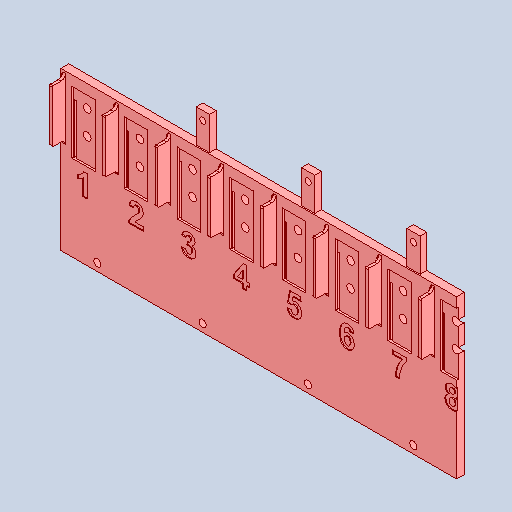
# Autodesk Inventor part: mainPlate
Saved by Autodesk Inventor 2024.3 (Build 283343000, 343)
## iProperties
Created: 2022-10-05
Part Number: mainPlate
Material: Generic
Document SubType Name: Modeling
Designer: Admin
Density: 1 g/cm^3
Appearance: Default(2)
x_d0: 1.000 ul
x_d1: 1.000 ul
x_d2: 1.000 ul
ref:MM:length: 9.750 in
ref:MMC:1: 0.150 in
ref:oring_gap: 0.018 in
ref:fsens:body:4: 0.228 in
ref:fsens:body:6: 0.203 in
ref:fsens:body:2: 0.328 in
ref:fsens:body:5: 1.073 in
ref:fsens:body:1: 1.200 in
ref:fsens:body:3: 0.610 in
ref:fsens:body:7: 0.125 in
ref:fsens:arc_cutout:1: 0.057 in
ref:fsens:arc_cutout:5: 0.550 in
ref:fsens:bottom_grooves:3: 0.940 in
ref:fsens:bottom_grooves:4: 0.058 in
ref:fsens:bottom_grooves:1: 0.155 in
ref:fsens:bottom_grooves:5: 0.500 in
ref:fsens:bottom_grooves:6: 0.040 in
ref:fsens:bottom_grooves:2: 0.473 in
ref:fsens:headerpins:2: 0.025 in
ref:fsens:headerpins:3: 0.100 in
ref:fsens:headerpins:4: 0.100 in
ref:fsens:headerpins:1: 0.025 in
ref:fsens:headerpins:5: 0.001 in
ref:fsens:arc_cutout:3: 0.325 in
ref:fsens:arc_cutout:4: 0.207 in
headerpins:extra_top_space: 0.125 in
headerpins:distance_to_clear_MM_and_MMC: 0.293 in
a_MP_thickness: 0.180 in
x_e0: 0.00 deg
x_e2: 0.00 deg
headerpins:wiggleroom:vertical: 0.491 in
bottom_groove:extra_top_space: 0.025 in
bottom_groove:distance_to_clear_MM_and_MMC: 0.293 in
bottom_groove:wiggleroom:vertical: 0.100 in
bottom_groove:extra_side_space_back: 0.010 in
fsens:bottom_groove:depth: 0.045 in
fsens:hole_diameter: 0.175 in
headerpins:extra_side_space: 0.005 in
p_num_patterns: 8.000 ul
p_pattern_spacing: 1.200 in
ref:fsens:arc_cutout:2: 0.110 in
ref:fsens:body:6:2: 0.203 in
ref:fsens:body:5:2: 1.073 in
ref:fsens:body:3:2: 0.610 in
ref:fsens:bottom_grooves:3:2: 0.940 in
ref:fsens:bottom_grooves:1:2: 0.155 in
ref:fsens:bottom_grooves:6:2: 0.040 in
ref:fsens:bottom_grooves:2:2: 0.473 in
bottom_groove:to_side: 0.250 in
ref:fsens_btm_groove_8th_one: 8.400 in
bottom_groove:to_side:2: 0.010 in
ref_440_throughhole: 0.165 in
MMscrews:to_top: 0.200 in
d133: 0.180 in
x_e3: 0.00 deg
MMscrews:through_hole:diameter: 0.140 in
MMscrews_popup_width: 0.300 in
ref:MMC:height: 0.150 in
ref:MM:width: 1.100 in
ref:MM:height: 0.800 in
d148: 0.018 in
MMC_to_top_of_MP: 0.030 in
d168: 0.029 in
d171: 0.029 in
x_e4: 0.00 deg
headerpins_space_for_PCB_female_headers: 0.150 in
headerpins:cutout_depth: 0.100 in
bottom_groove:extra_side_space_front: 0.020 in
fsens:front_wall:width: 0.085 in
fsens:front_wall:height: 0.300 in
x_e: 0.00 deg
d219: 0.025 in
d220: 0.025 in
d222: 0.100 in
d223: 0.025 in
numbers_width: 0.300 in
numbers_height: 0.500 in
numbers_space_between: 1.200 in
numbers_: 0.100 in
d244: 0.020 in
d245: 0.00 deg
d246: 0.300 in
d247: 0.500 in
d248: 0.100 in
d281: 0.020 in
d285: 0.165 in
d292: 2.400 in
d293: 2.400 in
d294: 2.400 in
d295: 3.975 in
d296: 0.025 in
d297: 0.175 in
d300: 9.016 in
d302: 0.00 deg
d303: 0.165 in
distance_to_clear_MM_and_MMC: 0.293 in
threadInsert_440:diameter: 0.175 in
bottom_groove:to_top: 0.230 in
d170: 0.035 in
a_mainManifold:x:length: 9.750 in
flowSensor:hole_insert:depth: 0.125 in
a_mainManifoldCover:y:height: 0.150 in
dsheet:side:z:1: 0.610 in
dsheet:front:x:1: 1.200 in
dsheet:front:x:4: 0.025 in
dsheet:front:x:2: 0.940 in
dsheet:front:x:3:1: 0.100 in
dsheet:top:x:3: 0.250 in
dsheet:top:x:4: 0.300 in
dsheet:top:x:2: 0.110 in
z_width: 0.328 in
headerpins_depth: 0.025 in
x_d47: 0.058 in
x_d51: 0.155 in
dsheet:front:x:3:2: 0.100 in
x_d53: 0.473 in
d55: 0.500 in
dsheet:top:x:1: 2.145 in
d64: 0.228 in
dsheet:side:z:4: 0.325 in
d65: 0.203 in
distance_between_MFCs: 1.200 in
a_mainManifold:y:height: 0.800 in
a_mainManifold:z:width: 1.100 in
Author: Admin
Autodesk Inventor part; units mm, degrees
ref_plane "YZ Plane" through (0, 0, 0) normal (1, 0, 0) x (0, 1, 0)
ref_plane "XZ Plane" through (0, 0, 0) normal (0, 1, 0) x (-1, 0, 0)
derived "main_manifold_8v_v02.ipt"
sketch "Sketch:MM: main inlet" plane through (0, 0, 0) normal (1, 0, 0) x (0, 1, 0)
  line L0 (20.32, 0) -> (0, 0)
  line L1 (0, 0) -> (0, -27.94)
  line L2 (0, -27.94) -> (20.32, -27.94)
  line L3 (20.32, -27.94) -> (20.32, 0)
  point P0 (13.97, -15.24)
sketch "Sketch:MM: prop valves" plane through (0, 0, -27.94) normal (0, 0, -1) x (-1, 0, 0)
  line L0 (-16.9926, 9.0678) -> (-24.9174, 9.0678) construction
  line L1 (-47.4726, 9.0678) -> (-55.3974, 9.0678) construction
  line L2 (-77.9526, 9.0678) -> (-85.8774, 9.0678) construction
  line L3 (-108.4326, 9.0678) -> (-116.3574, 9.0678) construction
  line L4 (-138.9126, 9.0678) -> (-146.8374, 9.0678) construction
  line L5 (-169.3926, 9.0678) -> (-177.3174, 9.0678) construction
  line L6 (-199.8726, 9.0678) -> (-207.7974, 9.0678) construction
  line L7 (-230.3526, 9.0678) -> (-238.2774, 9.0678) construction
  line L8 (-47.4726, 9.0678) -> (-51.435, 5.3848) construction
  line L9 (-16.9926, 9.0678) -> (-20.955, 5.3848) construction
  line L10 (-77.9526, 9.0678) -> (-81.915, 5.3848) construction
  line L11 (-169.3926, 9.0678) -> (-173.355, 5.3848) construction
  line L12 (-199.8726, 9.0678) -> (-203.835, 5.3848) construction
  line L13 (-230.3526, 9.0678) -> (-234.315, 5.3848) construction
  line L14 (-138.9126, 9.0678) -> (-142.875, 5.3848) construction
  line L15 (-108.4326, 9.0678) -> (-112.395, 5.3848) construction
  line L16 (-20.955, 12.5222) -> (-51.435, 12.5222) construction
  line L17 (-51.435, 12.5222) -> (-81.915, 12.5222) construction
  line L18 (-81.915, 12.5222) -> (-112.395, 12.5222) construction
  line L19 (-112.395, 12.5222) -> (-142.875, 12.5222) construction
  line L20 (-142.875, 12.5222) -> (-173.355, 12.5222) construction
  line L21 (-173.355, 12.5222) -> (-203.835, 12.5222) construction
  line L22 (-203.835, 12.5222) -> (-234.315, 12.5222) construction
  point P0 (0, 0)
  point P1 (0, 13.97)
sketch "Sketch:MM: prop valve cutout" plane through (0, 0, 0) normal (1, 0, 0) x (0, 1, 0)
  line L0 (20.32, -27.94) -> (20.32, 0)
  line L1 (0, -27.94) -> (20.32, -27.94)
  line L2 (20.32, -25.781) -> (16.256, -25.781)
  line L3 (16.256, -25.781) -> (16.256, -27.94)
  point P0 (0, 0)
  point P1 (12.5222, -27.94)
sketch "Sketch:MM: flow sensor" plane through (0, 0, -27.94) normal (0, -1, 0) x (1, 0, 0)
  line L0 (19.2278, 23.241) -> (22.6822, 23.241)
  line L1 (49.7078, 23.241) -> (53.1622, 23.241)
  line L2 (110.6678, 23.241) -> (114.1222, 23.241)
  line L3 (80.1878, 23.241) -> (83.6422, 23.241)
  line L4 (141.1478, 23.241) -> (144.6022, 23.241)
  line L5 (171.6278, 23.241) -> (175.0822, 23.241)
  line L6 (202.1078, 23.241) -> (205.5622, 23.241)
  line L7 (232.5878, 23.241) -> (236.0422, 23.241)
  line L8 (0, 27.94) -> (247.65, 27.94)
  point P0 (20.955, 23.241)
  point P1 (51.435, 23.241)
  point P2 (51.435, 23.241)
  point P3 (20.955, 23.241)
  point P4 (81.915, 23.241)
  point P5 (112.395, 23.241)
  point P6 (81.915, 23.241)
  point P7 (112.395, 23.241)
  point P8 (142.875, 23.241)
  point P9 (173.355, 23.241)
  point P10 (203.835, 23.241)
  point P11 (234.315, 23.241)
  point P12 (142.875, 23.241)
  point P13 (173.355, 23.241)
  point P14 (203.835, 23.241)
  point P15 (234.315, 23.241)
sketch "Sketch:MM: MMC screws" plane through (0, 20.32, 0) normal (0, 1, 0) x (1, 0, 0)
  line L0 (0, 0) -> (0, 27.94)
  line L1 (43.815, 4.699) -> (59.055, 4.699) construction
  line L2 (0, 0) -> (247.65, 0)
  line L3 (13.335, 4.699) -> (28.575, 4.699) construction
  line L4 (74.295, 4.699) -> (89.535, 4.699) construction
  line L5 (104.775, 4.699) -> (120.015, 4.699) construction
  line L6 (135.255, 4.699) -> (150.495, 4.699) construction
  line L7 (165.735, 4.699) -> (180.975, 4.699) construction
  line L8 (196.215, 4.699) -> (211.455, 4.699) construction
  line L9 (226.695, 4.699) -> (241.935, 4.699) construction
  point P0 (20.955, 4.699)
  point P1 (112.395, 4.699)
  point P2 (51.435, 4.699)
  point P3 (81.915, 4.699)
  point P4 (0, 25.781)
  point P5 (0, 25.781)
  point P6 (0, 25.781)
  point P7 (142.875, 4.699)
  point P8 (173.355, 4.699)
  point P9 (203.835, 4.699)
  point P10 (234.315, 4.699)
  point P11 (20.955, 4.699)
  point P12 (51.435, 4.699)
  point P13 (81.915, 4.699)
  point P14 (112.395, 4.699)
  point P15 (142.875, 4.699)
  point P16 (173.355, 4.699)
  point P17 (203.835, 4.699)
  point P18 (234.315, 4.699)
sketch "Sketch:MM: MP screws" plane through (0, 0, 0) normal (0, 0, 1) x (1, 0, 0)
  point P0 (0, 0)
  point P1 (5.08, 9.0678)
  point P2 (218.44, 9.0678)
  point P3 (96.52, 9.0678)
  point P4 (157.48, 9.0678)
sketch "Sketch:MM: mounting screws:1" plane through (0, 0, 0) normal (-1, 0, 0) x (0, 0, 1)
  line L0 (-27.94, 0) -> (-27.94, 16.256)
  line L1 (-21.59, 5.08) -> (-8.89, 5.08) construction
  point P0 (0, 0)
  point P1 (-15.24, 13.97)
  point P2 (-15.24, 5.08)
sketch "Sketch:MM: mounting screws:2" plane through (247.65, 0, 0) normal (1, 0, 0) x (0, 0, -1)
  point P0 (0, 0)
  point P1 (21.59, 5.08)
  point P2 (8.89, 5.08)
ref_plane "MM front face" through (0, 0, 0) normal (0, 0, 1) x (1, 0, 0)
derived "main_manifold_cover_1v_v02.ipt"
sketch "Sketch:MMC: base" plane through (0, 0, 0) normal (0, 1, 0) x (-1, 0, 0)
  line L0 (-9.779, -9.398) -> (-32.131, -9.398)
  line L1 (-32.131, -9.398) -> (-32.131, 0)
  line L2 (-32.131, 0) -> (-9.779, 0)
  line L3 (-9.779, 0) -> (-9.779, -9.398)
  point P0 (0, 0)
  point P1 (-43.815, -4.699)
  point P2 (-9.779, -4.699)
  point P3 (-13.335, -4.699)
  point P4 (-28.575, -4.699)
derived "Honeywell3000.ipt"
sketch "Sketch:ref: assembly:XY" plane through (0, 0, 0) normal (0, 0, 1) x (1, 0, 0)
  line L0 (0, 20.32) -> (0, 0) projected
  line L1 (0, 20.32) -> (247.65, 20.32)
  line L2 (247.65, 20.32) -> (247.65, 0)
  line L3 (247.65, 0) -> (0, 0)
  line L4 (9.779, 0) -> (32.131, 0) projected
  line L5 (9.779, -0.4572) -> (32.131, -0.4572)
  line L6 (32.131, -0.4572) -> (32.131, -4.2672)
  line L7 (32.131, -4.2672) -> (9.779, -4.2672)
  line L8 (9.779, -4.2672) -> (9.779, -0.4572)
  line L9 (18.0536, 3.175) -> (23.8564, 3.175)
  line L10 (23.8564, 3.175) -> (23.8564, -8.8265)
  line L11 (23.8564, -8.8265) -> (18.0536, -8.8265)
  line L12 (18.0536, -8.8265) -> (18.0536, 3.175)
  line L13 (17.7869, -8.8265) -> (26.1181, -8.8265)
  line L14 (26.1181, -8.8265) -> (26.1181, -39.3065)
  line L15 (26.1181, -39.3065) -> (17.7869, -39.3065)
  line L16 (17.7869, -39.3065) -> (17.7869, -8.8265)
  line L17 (26.1181, -8.8265) -> (33.2809, -8.8265)
  line L18 (33.2809, -8.8265) -> (33.2809, -39.3065)
  line L19 (33.2809, -39.3065) -> (26.1181, -39.3065)
  arc A0 (30.6647, -17.2745) -> (27.7691, -17.2745) centre (29.2169, -17.2745) ccw
  arc A1 (27.7691, -20.0685) -> (30.6647, -20.0685) centre (29.2169, -20.0685) ccw
  line L20 (27.7691, -20.0685) -> (27.7691, -17.2745)
  line L21 (30.6647, -20.0685) -> (30.6647, -17.2745)
  arc A2 (30.6647, -31.2445) -> (27.7691, -31.2445) centre (29.2169, -31.2445) ccw
  arc A3 (27.7691, -34.0385) -> (30.6647, -34.0385) centre (29.2169, -34.0385) ccw
  line L22 (27.7691, -34.0385) -> (27.7691, -31.2445)
  line L23 (30.6647, -34.0385) -> (30.6647, -31.2445)
  line L24 (29.2169, -17.2745) -> (29.2169, -20.0685) construction
  line L25 (29.2169, -31.2445) -> (29.2169, -34.0385) construction
  line L26 (21.971, -11.4935) -> (34.671, -11.4935)
  line L27 (34.671, -11.4935) -> (34.671, -12.9667)
  line L28 (34.671, -12.9667) -> (21.971, -12.9667)
  line L29 (21.971, -12.9667) -> (21.971, -11.4935)
  line L30 (21.971, -24.8412) -> (34.671, -24.8412)
  line L31 (34.671, -24.8412) -> (34.671, -26.3144)
  line L32 (34.671, -26.3144) -> (21.971, -26.3144)
  line L33 (21.971, -26.3144) -> (21.971, -24.8412)
  line L34 (21.971, -36.8427) -> (34.671, -36.8427)
  line L35 (34.671, -36.8427) -> (34.671, -35.3695)
  line L36 (34.671, -35.3695) -> (21.971, -35.3695)
  line L37 (21.971, -35.3695) -> (21.971, -36.8427)
  line L38 (21.971, -21.209) -> (22.606, -21.209)
  line L39 (22.606, -21.209) -> (22.606, -21.844)
  line L40 (22.606, -21.844) -> (21.971, -21.844)
  line L41 (21.971, -21.844) -> (21.971, -21.209)
  line L42 (21.971, -23.749) -> (22.606, -23.749)
  line L43 (22.606, -23.749) -> (22.606, -24.384)
  line L44 (22.606, -24.384) -> (21.971, -24.384)
  line L45 (21.971, -24.384) -> (21.971, -23.749)
  line L46 (21.971, -26.289) -> (22.606, -26.289)
  line L47 (22.606, -26.289) -> (22.606, -26.924)
  line L48 (22.606, -26.924) -> (21.971, -26.924)
  line L49 (21.971, -26.924) -> (21.971, -26.289)
  line L50 (231.4136, 3.175) -> (237.2164, 3.175)
  line L51 (237.2164, 3.175) -> (237.2164, -8.8265)
  line L52 (237.2164, -8.8265) -> (231.4136, -8.8265)
  line L53 (231.4136, -8.8265) -> (231.4136, 3.175)
  line L54 (231.1469, -8.8265) -> (239.4781, -8.8265)
  line L55 (239.4781, -8.8265) -> (239.4781, -39.3065)
  line L56 (239.4781, -39.3065) -> (231.1469, -39.3065)
  line L57 (231.1469, -39.3065) -> (231.1469, -8.8265)
  line L58 (239.4781, -8.8265) -> (246.6409, -8.8265)
  line L59 (246.6409, -8.8265) -> (246.6409, -39.3065)
  line L60 (246.6409, -39.3065) -> (239.4781, -39.3065)
  line L61 (235.331, -11.4935) -> (248.031, -11.4935)
  line L62 (248.031, -11.4935) -> (248.031, -12.9667)
  line L63 (248.031, -12.9667) -> (235.331, -12.9667)
  line L64 (235.331, -12.9667) -> (235.331, -11.4935)
  line L65 (235.331, -24.8412) -> (248.031, -24.8412)
  line L66 (248.031, -24.8412) -> (248.031, -26.3144)
  line L67 (248.031, -26.3144) -> (235.331, -26.3144)
  line L68 (235.331, -26.3144) -> (235.331, -24.8412)
  line L69 (235.331, -36.8427) -> (248.031, -36.8427)
  line L70 (248.031, -36.8427) -> (248.031, -35.3695)
  line L71 (248.031, -35.3695) -> (235.331, -35.3695)
  line L72 (235.331, -35.3695) -> (235.331, -36.8427)
  point P0 (20.955, 3.175)
  point P1 (20.955, 3.175)
  point P2 (17.7869, -24.0665)
  point P3 (17.7869, -24.0665)
  point P4 (20.955, 0)
  point P5 (29.2169, -32.6415)
  point P6 (29.2169, -18.6715)
  point P7 (29.2169, -18.6715)
  point P8 (34.671, -36.1061)
  point P9 (34.671, -36.1061)
  point P10 (34.671, -12.2301)
  point P11 (34.671, -12.2301)
  point P12 (22.606, -21.5265)
  point P13 (22.606, -24.0665)
  point P14 (22.606, -21.5265)
  point P15 (22.606, -24.0665)
  point P16 (22.606, -26.6065)
  point P17 (22.606, -26.6065)
  point P18 (234.315, 3.175)
  point P19 (234.315, 3.175)
  point P20 (231.1469, -24.0665)
  point P21 (231.1469, -24.0665)
  point P22 (248.031, -36.1061)
  point P23 (248.031, -36.1061)
  point P24 (248.031, -12.2301)
  point P25 (248.031, -12.2301)
  point P26 (234.315, 0)
  constraints: 142 end point, 44 perpendicular, 21 equal length, 16 coincident, 15 collinear, 14 vertical alignment, 13 midpoint, 8 parallel, 8 point on circle, 8 tangent, 6 horizontal, 5 horizontal alignment, 4 centre point, 4 point on line, 3 equal radius, 2 vertical, 10 other
sketch "x_Sketch:ref: assembly:YZ" plane through (0, 0, 0) normal (1, 0, 0) x (0, 1, 0)
  line L0 (-0.4572, 27.2034) -> (-4.2672, 27.2034)
  line L1 (-4.2672, 27.2034) -> (-4.2672, 17.8054)
  line L2 (-4.2672, 17.8054) -> (-0.4572, 17.8054)
  line L3 (-0.4572, 17.8054) -> (-0.4572, 27.2034)
  line L4 (0, -9.398) -> (0, 0) construction
  line L5 (20.32, 27.2034) -> (0, 27.2034)
  line L6 (0, 27.2034) -> (0, -0.7366)
  line L7 (0, -0.7366) -> (20.32, -0.7366)
  line L8 (20.32, -0.7366) -> (20.32, 27.2034)
  point P0 (0, 0)
  dimension "d148" = 0.4572
  dimension "d168" = 0.7366
  constraints: 16 end point, 6 perpendicular, 2 horizontal, 2 horizontal alignment, 1 collinear, 1 parallel, 1 point on line, 1 vertical alignment
  measures "d148" distance between parallel lines of L3 L6
  measures "d168" distance from line of point (0, 0) L7
sketch "Sketch:MP:fSens header pins" plane through (0, 0, 0) normal (0, 0, 1) x (1, 0, 0)
  line L0 (17.7869, -39.3065) -> (17.7869, -8.8265) construction
  line L1 (33.2809, -8.8265) -> (33.2809, -39.3065) construction
  line L2 (26.1181, -39.3065) -> (17.7869, -39.3065) construction
  line L3 (33.2809, -39.3065) -> (26.1181, -39.3065) construction
  line L4 (26.1181, -8.8265) -> (33.2809, -8.8265) construction
  line L5 (17.7869, -8.8265) -> (26.1181, -8.8265) construction
  line L6 (30.6647, -20.0685) -> (30.6647, -17.2745) construction
  arc A0 (30.6647, -17.2745) -> (27.7691, -17.2745) centre (29.2169, -17.2745) ccw construction
  line L7 (27.7691, -20.0685) -> (27.7691, -17.2745) construction
  arc A1 (27.7691, -20.0685) -> (30.6647, -20.0685) centre (29.2169, -20.0685) ccw construction
  arc A2 (30.6647, -31.2445) -> (27.7691, -31.2445) centre (29.2169, -31.2445) ccw construction
  line L8 (30.6647, -34.0385) -> (30.6647, -31.2445) construction
  arc A3 (27.7691, -34.0385) -> (30.6647, -34.0385) centre (29.2169, -34.0385) ccw construction
  line L9 (27.7691, -34.0385) -> (27.7691, -31.2445) construction
  line L10 (22.606, -26.924) -> (21.971, -26.924) construction
  line L11 (21.971, -26.924) -> (21.971, -26.289) construction
  line L12 (22.606, -26.289) -> (22.606, -26.924) construction
  line L13 (21.971, -26.289) -> (22.606, -26.289) construction
  line L14 (22.606, -24.384) -> (21.971, -24.384) construction
  line L15 (22.606, -23.749) -> (22.606, -24.384) construction
  line L16 (21.971, -24.384) -> (21.971, -23.749) construction
  line L17 (21.971, -23.749) -> (22.606, -23.749) construction
  line L18 (22.606, -21.844) -> (21.971, -21.844) construction
  line L19 (22.606, -21.209) -> (22.606, -21.844) construction
  line L20 (21.971, -21.844) -> (21.971, -21.209) construction
  line L21 (21.971, -21.209) -> (22.606, -21.209) construction
  line L22 (21.971, -11.4935) -> (34.671, -11.4935) construction
  line L23 (21.971, -12.9667) -> (21.971, -11.4935) construction
  line L24 (34.671, -12.9667) -> (21.971, -12.9667) construction
  line L25 (34.671, -11.4935) -> (34.671, -12.9667) construction
  line L26 (34.671, -26.3144) -> (21.971, -26.3144) construction
  line L27 (21.971, -24.8412) -> (34.671, -24.8412) construction
  line L28 (34.671, -24.8412) -> (34.671, -26.3144) construction
  line L29 (21.971, -26.3144) -> (21.971, -24.8412) construction
  line L30 (34.671, -35.3695) -> (21.971, -35.3695) construction
  line L31 (21.971, -35.3695) -> (21.971, -36.8427) construction
  line L32 (21.971, -36.8427) -> (34.671, -36.8427) construction
  line L33 (34.671, -36.8427) -> (34.671, -35.3695) construction
  line L34 (21.844, -18.034) -> (22.733, -18.034)
  line L35 (22.733, -18.034) -> (22.733, -46.8249)
  line L36 (22.733, -46.8249) -> (21.844, -46.8249)
  line L37 (21.844, -46.8249) -> (21.844, -18.034)
  line L38 (22.733, -34.3662) -> (21.844, -34.3662) construction
  line L39 (20.3835, -18.034) -> (24.1935, -18.034)
  line L40 (24.1935, -18.034) -> (24.1935, -46.8249)
  line L41 (24.1935, -46.8249) -> (20.3835, -46.8249)
  line L42 (20.3835, -46.8249) -> (20.3835, -18.034)
  point P0 (0, 0)
  point P1 (22.2885, -18.034)
  point P2 (22.2885, -21.209)
  point P3 (22.2885, -18.034)
  dimension "headerpins_space_for_PCB_female_headers" = 3.81
  constraints: 18 end point, 7 perpendicular, 4 parallel, 3 midpoint, 2 collinear, 2 point on line, 1 coincident, 1 horizontal, 1 vertical alignment
  measures "headerpins_space_for_PCB_female_headers" distance of L39.start L39.end
sketch "Sketch:MP:fSens bottom groove" plane through (0, 0, 0) normal (0, 0, 1) x (1, 0, 0)
  line L0 (21.971, -11.4935) -> (34.671, -11.4935) construction
  line L1 (21.971, -12.9667) -> (21.971, -11.4935) construction
  line L2 (34.671, -12.9667) -> (21.971, -12.9667) construction
  line L3 (34.671, -11.4935) -> (34.671, -12.9667) construction
  line L4 (34.671, -24.8412) -> (34.671, -26.3144) construction
  line L5 (21.971, -24.8412) -> (34.671, -24.8412) construction
  line L6 (34.671, -26.3144) -> (21.971, -26.3144) construction
  line L7 (21.971, -26.3144) -> (21.971, -24.8412) construction
  line L8 (34.671, -35.3695) -> (21.971, -35.3695) construction
  line L9 (34.671, -36.8427) -> (34.671, -35.3695) construction
  line L10 (21.971, -36.8427) -> (34.671, -36.8427) construction
  line L11 (21.971, -35.3695) -> (21.971, -36.8427) construction
  line L12 (21.463, -10.8585) -> (34.925, -10.8585)
  line L13 (34.925, -10.8585) -> (34.925, -46.8249)
  line L14 (34.925, -46.8249) -> (21.463, -46.8249)
  line L15 (21.463, -46.8249) -> (21.463, -10.8585)
  line L16 (34.925, -44.2849) -> (21.463, -44.2849) construction
  line L17 (22.733, -18.034) -> (22.733, -46.8249) construction
  line L18 (21.844, -18.034) -> (22.733, -18.034) construction
  line L19 (21.844, -46.8249) -> (21.844, -18.034) construction
  line L20 (22.733, -46.8249) -> (21.844, -46.8249) construction
  point P0 (0, 0)
  point P1 (28.321, -11.4935)
  point P2 (28.194, -10.8585)
  constraints: 8 end point, 4 parallel, 3 horizontal, 2 midpoint, 2 perpendicular, 1 point on line, 1 vertical, 4 other
sketch "Sketch:MP:fSens front wall" plane through (0, 0, 0) normal (0, 0, 1) x (1, 0, 0)
  line L0 (15.6279, -8.8265) -> (17.7869, -8.8265)
  line L1 (17.7869, -8.8265) -> (17.7869, -39.3065)
  line L2 (17.7869, -39.3065) -> (15.6279, -39.3065)
  line L3 (15.6279, -39.3065) -> (15.6279, -8.8265)
  line L4 (17.7869, -39.3065) -> (17.7869, -8.8265) construction
  line L5 (17.7869, -8.8265) -> (26.1181, -8.8265) construction
  line L6 (26.1181, -39.3065) -> (17.7869, -39.3065) construction
  point P0 (0, 0)
  constraints: 8 end point, 3 collinear, 2 parallel, 1 horizontal, 1 horizontal alignment, 1 perpendicular
sketch "Sketch:MP: VH holes" plane through (0, 0, 0) normal (0, 0, 1) x (1, 0, 0)
  line L0 (36.195, -91.8972) -> (97.155, -91.8972)
  line L1 (97.155, -91.8972) -> (158.115, -91.8972)
  line L2 (158.115, -91.8972) -> (219.075, -91.8972)
  point P0 (0, 0)
  point P1 (5.08, 9.0678)
  point P2 (96.52, 9.0678)
  point P3 (157.48, 9.0678)
  point P4 (218.44, 9.0678)
  dimension "d292" = 60.96
  dimension "d293" = 60.96
  dimension "d294" = 60.96
  dimension "d295" = 100.965
  dimension "d296" = 0.635
  constraints: 6 end point, 4 coincident, 3 horizontal alignment
  measures "d292" distance of L0.start L0.end
  measures "d293" distance of L0.end L1.end
  measures "d294" distance of L1.end L2.end
  measures "d295" vertical distance of point (219.075, -91.897) point (218.44, 9.068)
  measures "d296" horizontal distance of point (219.075, -91.897) point (218.44, 9.068)
sketch "Sketch:MP:base" plane through (0, 0, 0) normal (0, 0, 1) x (1, 0, 0)
  line L0 (15.113, -5.0292) -> (248.539, -5.0292)
  line L1 (248.539, -5.0292) -> (248.539, -96.3422)
  line L2 (248.539, -96.3422) -> (15.113, -96.3422)
  line L3 (15.113, -96.3422) -> (15.113, -5.0292)
  line L4 (21.463, -10.8585) -> (34.925, -10.8585) construction
  line L5 (21.463, -46.8249) -> (21.463, -10.8585) construction
  line L6 (34.925, -10.8585) -> (34.925, -46.8249) construction
  line L7 (34.925, -46.8249) -> (21.463, -46.8249) construction
  line L8 (234.823, -10.8585) -> (248.285, -10.8585) construction
  line L9 (248.285, -10.8585) -> (248.285, -46.8249) construction
  line L10 (248.285, -46.8249) -> (234.823, -46.8249) construction
  line L11 (234.823, -46.8249) -> (234.823, -10.8585) construction
  line L12 (247.65, 0) -> (0, 0) construction
  line L13 (32.131, -4.2672) -> (9.779, -4.2672) construction
  line L14 (9.779, -4.2672) -> (9.779, -0.4572) construction
  line L15 (9.779, -0.4572) -> (32.131, -0.4572) construction
  line L16 (32.131, -0.4572) -> (32.131, -4.2672) construction
  point P0 (36.195, -91.8972)
  point P1 (97.155, -91.8972)
  point P2 (158.115, -91.8972)
  point P3 (219.075, -91.8972)
  dimension "MMC_to_top_of_MP" = 0.762
  dimension "d170" = 0.889
  dimension "d297" = 4.445
  constraints: 16 end point, 4 equal length, 4 parallel, 2 perpendicular, 1 collinear
  measures "MMC_to_top_of_MP" distance between parallel lines of L0 L13
  measures "d170" distance from line of L1 L12.start
  measures "d297" distance from line of L2 point (36.195, -91.897)
sketch "Sketch:MP: MM screws" plane through (0, 0, 0) normal (0, 0, 1) x (1, 0, 0)
  line L0 (0, 20.32) -> (247.65, 20.32) construction
  line L1 (247.65, 20.32) -> (247.65, 0) construction
  line L2 (0, 20.32) -> (0, 0) construction
  line L3 (247.65, 0) -> (0, 0) construction
  line L4 (15.113, -96.3422) -> (15.113, -5.0292) projected
  line L5 (15.113, -5.0292) -> (248.539, -5.0292) projected
  line L6 (248.539, -5.0292) -> (248.539, -96.3422) projected
  line L7 (92.71, -5.0292) -> (92.71, 14.1478)
  line L8 (92.71, 14.1478) -> (100.33, 14.1478)
  line L9 (100.33, 14.1478) -> (100.33, -5.0292)
  line L10 (153.67, -5.0292) -> (153.67, 14.1478)
  line L11 (153.67, 14.1478) -> (161.29, 14.1478)
  line L12 (161.29, 14.1478) -> (161.29, -5.0292)
  line L13 (214.63, -5.0292) -> (214.63, 14.1478)
  line L14 (214.63, 14.1478) -> (222.25, 14.1478)
  line L15 (222.25, 14.1478) -> (222.25, -5.0292)
  circle A0 centre (96.52, 9.0678) radius 2.0955 construction
  point P0 (5.08, 9.0678)
  point P1 (157.48, 9.0678)
  point P2 (218.44, 9.0678)
  point P3 (96.52, 14.1478)
  point P4 (157.48, 14.1478)
  point P5 (218.44, 14.1478)
  dimension "ref_440_throughhole" = 4.191
  dimension "MMscrews_popup_width" = 7.62
  constraints: 18 end point, 9 perpendicular, 6 point on line, 4 collinear, 3 midpoint, 3 vertical alignment, 1 centre point, 1 coincident, 1 other
  measures "ref_440_throughhole" diameter of A0
  measures "MMscrews_popup_width" distance of L7.end L8.end
sketch "Sketch:MP:numbers_front" plane through (0, 0, 0) normal (0, 0, 1) x (1, 0, 0)
  line L0 (24.384, -50.1583) -> (32.004, -50.1583) construction
  line L1 (32.004, -50.1583) -> (32.004, -62.8583) construction
  line L2 (32.004, -62.8583) -> (24.384, -62.8583) construction
  line L3 (24.384, -62.8583) -> (24.384, -50.1583) construction
  line L4 (54.864, -50.1583) -> (62.484, -50.1583) construction
  line L5 (62.484, -50.1583) -> (62.484, -62.8583) construction
  line L6 (62.484, -62.8583) -> (54.864, -62.8583) construction
  line L7 (54.864, -62.8583) -> (54.864, -50.1583) construction
  line L8 (85.344, -50.1583) -> (92.964, -50.1583) construction
  line L9 (92.964, -50.1583) -> (92.964, -62.8583) construction
  line L10 (92.964, -62.8583) -> (85.344, -62.8583) construction
  line L11 (85.344, -62.8583) -> (85.344, -50.1583) construction
  line L12 (115.824, -50.1583) -> (123.444, -50.1583) construction
  line L13 (123.444, -50.1583) -> (123.444, -62.8583) construction
  line L14 (123.444, -62.8583) -> (115.824, -62.8583) construction
  line L15 (115.824, -62.8583) -> (115.824, -50.1583) construction
  line L16 (146.304, -50.1583) -> (153.924, -50.1583) construction
  line L17 (153.924, -50.1583) -> (153.924, -62.8583) construction
  line L18 (153.924, -62.8583) -> (146.304, -62.8583) construction
  line L19 (146.304, -62.8583) -> (146.304, -50.1583) construction
  line L20 (176.784, -50.1583) -> (184.404, -50.1583) construction
  line L21 (184.404, -50.1583) -> (184.404, -62.8583) construction
  line L22 (184.404, -62.8583) -> (176.784, -62.8583) construction
  line L23 (176.784, -62.8583) -> (176.784, -50.1583) construction
  line L24 (207.264, -50.1583) -> (214.884, -50.1583) construction
  line L25 (214.884, -50.1583) -> (214.884, -62.8583) construction
  line L26 (214.884, -62.8583) -> (207.264, -62.8583) construction
  line L27 (207.264, -62.8583) -> (207.264, -50.1583) construction
  line L28 (237.744, -50.1583) -> (245.364, -50.1583) construction
  line L29 (245.364, -50.1583) -> (245.364, -62.8583) construction
  line L30 (245.364, -62.8583) -> (237.744, -62.8583) construction
  line L31 (237.744, -62.8583) -> (237.744, -50.1583) construction
  line L32 (28.194, -65.3983) -> (58.674, -65.3983) construction
  line L33 (58.674, -65.3983) -> (89.154, -65.3983) construction
  line L34 (89.154, -65.3983) -> (119.634, -65.3983) construction
  line L35 (119.634, -65.3983) -> (150.114, -65.3983) construction
  line L36 (150.114, -65.3983) -> (180.594, -65.3983) construction
  line L37 (180.594, -65.3983) -> (211.074, -65.3983) construction
  line L38 (211.074, -65.3983) -> (241.554, -65.3983) construction
  line L39 (21.463, -10.8585) -> (34.925, -10.8585) construction
  line L40 (34.925, -10.8585) -> (34.925, -46.8249) construction
  line L41 (21.463, -46.8249) -> (21.463, -10.8585) construction
  line L42 (34.925, -46.8249) -> (21.463, -46.8249) construction
  line L43 (30.251, -62.9067) -> (27.8116, -62.9067)
  line L44 (27.8116, -62.9067) -> (27.8116, -53.7398)
  spline S0 degree 2 poles (27.8116, -53.7398) (26.4758, -54.9789) (24.6657, -55.579) knots 0 0 0 1 1 1
  line L45 (24.6657, -55.579) -> (24.6657, -53.372)
  spline S1 degree 2 poles (24.6657, -53.372) (25.624, -53.0622) (27.86, -51.3199) (28.2763, -50.1583) knots 0 0 0 1 2 2 2
  line L46 (28.2763, -50.1583) -> (30.251, -50.1583)
  line L47 (30.251, -50.1583) -> (30.251, -62.9067)
  line L48 (62.7153, -60.6416) -> (62.7153, -62.9067)
  line L49 (62.7153, -62.9067) -> (54.1874, -62.9067)
  spline S2 degree 2 poles (54.1874, -62.9067) (54.3229, -61.6289) (55.7071, -59.3348) (57.7593, -57.4375) knots 0 0 0 1 2 2 2
  spline S3 degree 2 poles (57.7593, -57.4375) (59.4048, -55.9081) (59.7727, -55.3564) knots 0 0 0 1 1 1
  spline S4 degree 2 poles (59.7727, -55.3564) (60.276, -54.6013) (60.276, -53.8657) knots 0 0 0 1 1 1
  spline S5 degree 2 poles (60.276, -53.8657) (60.276, -53.0526) (59.4048, -52.1814) (58.6304, -52.1814) knots 0 0 0 1 2 2 2
  spline S6 degree 2 poles (58.6304, -52.1814) (57.8754, -52.1814) (56.9752, -53.101) (56.9074, -54.1657) knots 0 0 0 1 2 2 2
  line L50 (56.9074, -54.1657) -> (54.4778, -53.9238)
  spline S7 degree 2 poles (54.4778, -53.9238) (54.6907, -51.9103) (56.9752, -50.1583) (58.6885, -50.1583) knots 0 0 0 1 2 2 2
  spline S8 degree 2 poles (58.6885, -50.1583) (60.5664, -50.1583) (62.7153, -52.1814) (62.7153, -53.6914) knots 0 0 0 1 2 2 2
  spline S9 degree 2 poles (62.7153, -53.6914) (62.7153, -54.5433) (62.1055, -56.092) (61.4376, -56.9439) knots 0 0 0 1 2 2 2
  spline S10 degree 2 poles (61.4376, -56.9439) (60.9923, -57.5053) (58.6885, -59.6155) (58.069, -60.3125) (57.8851, -60.6416) knots 0 0 0 1 2 3 3 3
  line L51 (57.8851, -60.6416) -> (62.7153, -60.6416)
  line L52 (84.89, -59.5284) -> (87.2422, -59.238)
  spline S11 degree 2 poles (87.2422, -59.238) (87.3584, -60.1382) (88.3457, -61.0965) (89.0427, -61.0965) knots 0 0 0 1 2 2 2
  spline S12 degree 2 poles (89.0427, -61.0965) (89.7977, -61.0965) (90.8238, -59.9543) (90.8238, -58.9863) knots 0 0 0 1 2 2 2
  spline S13 degree 2 poles (90.8238, -58.9863) (90.8238, -58.0667) (89.8461, -56.9923) (89.1395, -56.9923) knots 0 0 0 1 2 2 2
  spline S14 degree 2 poles (89.1395, -56.9923) (88.6748, -56.9923) (88.0263, -57.1762) knots 0 0 0 1 1 1
  line L53 (88.0263, -57.1762) -> (88.2973, -55.1918)
  spline S15 degree 2 poles (88.2973, -55.1918) (89.2847, -55.2209) (90.3204, -54.3109) (90.3204, -53.5559) knots 0 0 0 1 2 2 2
  spline S16 degree 2 poles (90.3204, -53.5559) (90.3204, -52.917) (89.5557, -52.162) (88.9265, -52.162) knots 0 0 0 1 2 2 2
  spline S17 degree 2 poles (88.9265, -52.162) (88.2973, -52.162) (87.4165, -53.0235) (87.3197, -53.856) knots 0 0 0 1 2 2 2
  line L54 (87.3197, -53.856) -> (85.0739, -53.4785)
  spline S18 degree 2 poles (85.0739, -53.4785) (85.3062, -52.3266) (86.2549, -50.9423) (87.9392, -50.1583) (88.9943, -50.1583) knots 0 0 0 1 2 3 3 3
  spline S19 degree 2 poles (88.9943, -50.1583) (90.7851, -50.1583) (91.8692, -51.3005) knots 0 0 0 1 1 1
  spline S20 degree 2 poles (91.8692, -51.3005) (92.7598, -52.2298) (92.7598, -53.4107) knots 0 0 0 1 1 1
  spline S21 degree 2 poles (92.7598, -53.4107) (92.7598, -55.0757) (90.9303, -56.0727) knots 0 0 0 1 1 1
  spline S22 degree 2 poles (90.9303, -56.0727) (92.0241, -56.305) (93.3212, -57.9409) (93.3212, -59.0928) knots 0 0 0 1 2 2 2
  spline S23 degree 2 poles (93.3212, -59.0928) (93.3212, -60.7674) (90.8819, -63.1196) (89.062, -63.1196) knots 0 0 0 1 2 2 2
  spline S24 degree 2 poles (89.062, -63.1196) (87.339, -63.1196) (85.0739, -61.1353) (84.89, -59.5284) knots 0 0 0 1 2 2 2
  line L55 (120.2293, -62.9067) -> (120.2293, -60.3512)
  line L56 (120.2293, -60.3512) -> (115.0312, -60.3512)
  line L57 (115.0312, -60.3512) -> (115.0312, -58.2313)
  line L58 (115.0312, -58.2313) -> (120.5391, -50.1583)
  line L59 (120.5391, -50.1583) -> (122.5815, -50.1583)
  line L60 (122.5815, -50.1583) -> (122.5815, -58.2216)
  line L61 (122.5815, -58.2216) -> (124.1593, -58.2216)
  line L62 (124.1593, -58.2216) -> (124.1593, -60.3512)
  line L63 (124.1593, -60.3512) -> (122.5815, -60.3512)
  line L64 (122.5815, -60.3512) -> (122.5815, -62.9067)
  line L65 (122.5815, -62.9067) -> (120.2293, -62.9067)
  line L66 (120.2293, -58.2216) -> (120.2293, -53.8754)
  line L67 (120.2293, -53.8754) -> (117.306, -58.2216)
  line L68 (117.306, -58.2216) -> (120.2293, -58.2216)
  line L69 (145.9662, -59.4316) -> (148.3958, -59.1799)
  spline S25 degree 2 poles (148.3958, -59.1799) (148.5023, -60.0027) (149.5187, -60.961) (150.1866, -60.961) knots 0 0 0 1 2 2 2
  spline S26 degree 2 poles (150.1866, -60.961) (150.9513, -60.961) (152.0064, -59.722) (152.0064, -58.4636) knots 0 0 0 1 2 2 2
  spline S27 degree 2 poles (152.0064, -58.4636) (152.0064, -57.2923) (150.9513, -56.1211) (150.1092, -56.1211) knots 0 0 0 1 2 2 2
  spline S28 degree 2 poles (150.1092, -56.1211) (149.0637, -56.1211) (148.2313, -57.0504) knots 0 0 0 1 1 1
  line L70 (148.2313, -57.0504) -> (146.2566, -56.76)
  line L71 (146.2566, -56.76) -> (147.5053, -50.1583)
  line L72 (147.5053, -50.1583) -> (153.9521, -50.1583)
  line L73 (153.9521, -50.1583) -> (153.9521, -52.433)
  line L74 (153.9521, -52.433) -> (149.3541, -52.433)
  line L75 (149.3541, -52.433) -> (148.9669, -54.5917)
  spline S29 degree 2 poles (148.9669, -54.5917) (149.78, -54.1851) (150.6319, -54.1851) knots 0 0 0 1 1 1
  spline S30 degree 2 poles (150.6319, -54.1851) (152.2581, -54.1851) (154.5135, -56.547) (154.5135, -58.4249) knots 0 0 0 1 2 2 2
  spline S31 degree 2 poles (154.5135, -58.4249) (154.5135, -59.993) (153.6036, -61.2224) knots 0 0 0 1 1 1
  spline S32 degree 2 poles (153.6036, -61.2224) (152.3646, -62.9067) (150.1576, -62.9067) knots 0 0 0 1 1 1
  spline S33 degree 2 poles (150.1576, -62.9067) (148.4055, -62.9067) (146.1791, -61.0191) (145.9662, -59.4316) knots 0 0 0 1 2 2 2
  line L76 (184.6644, -53.3139) -> (182.3122, -53.5753)
  spline S34 degree 2 poles (182.3122, -53.5753) (182.2251, -52.8493) (181.4991, -52.162) (180.9183, -52.162) knots 0 0 0 1 2 2 2
  spline S35 degree 2 poles (180.9183, -52.162) (180.1439, -52.162) (179.0791, -53.5462) (178.9436, -55.7339) knots 0 0 0 1 2 2 2
  spline S36 degree 2 poles (178.9436, -55.7339) (179.8438, -54.6594) (181.199, -54.6594) knots 0 0 0 1 1 1
  spline S37 degree 2 poles (181.199, -54.6594) (182.7187, -54.6594) (184.8967, -56.9826) (184.8967, -58.8121) knots 0 0 0 1 2 2 2
  spline S38 degree 2 poles (184.8967, -58.8121) (184.8967, -60.7674) (182.6123, -63.1196) (180.8215, -63.1196) knots 0 0 0 1 2 2 2
  spline S39 degree 2 poles (180.8215, -63.1196) (178.8952, -63.1196) (176.4171, -60.1286) (176.4171, -56.7309) knots 0 0 0 1 2 2 2
  spline S40 degree 2 poles (176.4171, -56.7309) (176.4171, -53.2365) (179.0017, -50.1583) (181.0635, -50.1583) knots 0 0 0 1 2 2 2
  spline S41 degree 2 poles (181.0635, -50.1583) (182.5058, -50.1583) (184.403, -51.7748) (184.6644, -53.3139) knots 0 0 0 1 2 2 2
  spline S42 degree 2 poles (179.1469, -58.6185) (179.1469, -59.8091) (180.2407, -61.0965) (180.9376, -61.0965) knots 0 0 0 1 2 2 2
  spline S43 degree 2 poles (180.9376, -61.0965) (181.6152, -61.0965) (182.5155, -60.0414) (182.5155, -58.8411) knots 0 0 0 1 2 2 2
  spline S44 degree 2 poles (182.5155, -58.8411) (182.5155, -57.6021) (181.5475, -56.4502) (180.8215, -56.4502) knots 0 0 0 1 2 2 2
  spline S45 degree 2 poles (180.8215, -56.4502) (180.1148, -56.4502) (179.1469, -57.5537) (179.1469, -58.6185) knots 0 0 0 1 2 2 2
  line L77 (206.8971, -52.4234) -> (206.8971, -50.1583)
  line L78 (206.8971, -50.1583) -> (215.2218, -50.1583)
  line L79 (215.2218, -50.1583) -> (215.2218, -51.9297)
  spline S46 degree 2 poles (215.2218, -51.9297) (214.1958, -52.9461) (212.0662, -56.7406) (210.9433, -61.0094) (210.953, -62.6937) knots 0 0 0 1 2 3 3 3
  line L80 (210.953, -62.6937) -> (208.6008, -62.6937)
  spline S47 degree 2 poles (208.6008, -62.6937) (208.6589, -60.0608) (210.7207, -54.582) (212.434, -52.4234) knots 0 0 0 1 2 2 2
  line L81 (212.434, -52.4234) -> (206.8971, -52.4234)
  spline S48 degree 2 poles (239.4583, -56.0533) (238.5194, -55.6564) (237.6578, -54.2625) (237.6578, -53.4301) knots 0 0 0 1 2 2 2
  spline S49 degree 2 poles (237.6578, -53.4301) (237.6578, -52.0071) (239.6422, -50.1583) (241.4717, -50.1583) knots 0 0 0 1 2 2 2
  spline S50 degree 2 poles (241.4717, -50.1583) (243.2819, -50.1583) (245.2856, -52.0071) (245.2856, -53.4301) knots 0 0 0 1 2 2 2
  spline S51 degree 2 poles (245.2856, -53.4301) (245.2856, -54.3109) (244.366, -55.6855) (243.5335, -56.0533) knots 0 0 0 1 2 2 2
  spline S52 degree 2 poles (243.5335, -56.0533) (244.5886, -56.4792) (245.6921, -58.1055) (245.6921, -59.1702) knots 0 0 0 1 2 2 2
  spline S53 degree 2 poles (245.6921, -59.1702) (245.6921, -60.932) (243.4464, -63.1293) (241.5879, -63.1293) knots 0 0 0 1 2 2 2
  spline S54 degree 2 poles (241.5879, -63.1293) (239.8552, -63.1293) (238.7033, -62.2194) knots 0 0 0 1 1 1
  spline S55 degree 2 poles (238.7033, -62.2194) (237.3384, -61.1449) (237.3384, -59.2767) knots 0 0 0 1 1 1
  spline S56 degree 2 poles (237.3384, -59.2767) (237.3384, -58.241) (238.3645, -56.518) (239.4583, -56.0533) knots 0 0 0 1 2 2 2
  spline S57 degree 2 poles (239.739, -59.0444) (239.739, -60.0511) (240.7651, -61.174) (241.5395, -61.174) knots 0 0 0 1 2 2 2
  spline S58 degree 2 poles (241.5395, -61.174) (242.2945, -61.174) (243.2819, -60.0898) (243.2819, -59.0638) knots 0 0 0 1 2 2 2
  spline S59 degree 2 poles (243.2819, -59.0638) (243.2819, -58.1732) (242.2752, -57.0891) (241.5104, -57.0891) knots 0 0 0 1 2 2 2
  spline S60 degree 2 poles (241.5104, -57.0891) (240.6102, -57.0891) (239.739, -58.3184) (239.739, -59.0444) knots 0 0 0 1 2 2 2
  spline S61 degree 2 poles (239.9617, -53.6043) (239.9617, -54.3303) (240.7844, -55.1434) (241.4717, -55.1434) knots 0 0 0 1 2 2 2
  spline S62 degree 2 poles (241.4717, -55.1434) (242.1687, -55.1434) (243.0011, -54.3206) (243.0011, -53.5946) knots 0 0 0 1 2 2 2
  spline S63 degree 2 poles (243.0011, -53.5946) (243.0011, -52.917) (242.1784, -52.0943) (241.5008, -52.0943) knots 0 0 0 1 2 2 2
  spline S64 degree 2 poles (241.5008, -52.0943) (240.7941, -52.0943) (239.9617, -52.9267) (239.9617, -53.6043) knots 0 0 0 1 2 2 2
  point P0 (0, 0)
  point P1 (28.194, -62.8583)
  point P2 (58.674, -62.8583)
  point P3 (89.154, -62.8583)
  point P4 (119.634, -62.8583)
  point P5 (150.114, -62.8583)
  point P6 (180.594, -62.8583)
  point P7 (211.074, -62.8583)
  point P8 (241.554, -62.8583)
  point P9 (28.194, -46.8249)
  point P10 (28.194, -50.1583)
  dimension "numbers_width" = 7.62
  dimension "numbers_height" = 12.7
  dimension "numbers_space_between" = 30.48
  dimension "numbers_" = 2.54
  constraints: 20 equal length, 14 end point, 13 collinear, 10 midpoint, 9 horizontal, 9 vertical alignment, 16 other
  measures "numbers_width" distance of L0.start L0.end
  measures "numbers_height" distance of L2.end L0.start
  measures "numbers_space_between" distance of L32.start L32.end
  measures "numbers_" distance between parallel lines of L32 L2
ref_plane "Work Plane1" through (0, 0, 2.54) normal (0, 0, -1) x (-1, 0, 0)
sketch "Sketch:MP:numbers_back" plane through (0, 0, 2.54) normal (0, 0, -1) x (-1, 0, 0)
  line L0 (-32.004, -50.1583) -> (-24.384, -50.1583) construction
  line L1 (-24.384, -50.1583) -> (-24.384, -62.8583) construction
  line L2 (-24.384, -62.8583) -> (-32.004, -62.8583) construction
  line L3 (-32.004, -62.8583) -> (-32.004, -50.1583) construction
  line L4 (-62.484, -50.1583) -> (-54.864, -50.1583) construction
  line L5 (-54.864, -50.1583) -> (-54.864, -62.8583) construction
  line L6 (-54.864, -62.8583) -> (-62.484, -62.8583) construction
  line L7 (-62.484, -62.8583) -> (-62.484, -50.1583) construction
  line L8 (-92.964, -62.8583) -> (-92.964, -50.1583) construction
  line L9 (-92.964, -50.1583) -> (-85.344, -50.1583) construction
  line L10 (-85.344, -50.1583) -> (-85.344, -62.8583) construction
  line L11 (-85.344, -62.8583) -> (-92.964, -62.8583) construction
  line L12 (-123.444, -62.8583) -> (-123.444, -50.1583) construction
  line L13 (-123.444, -50.1583) -> (-115.824, -50.1583) construction
  line L14 (-115.824, -50.1583) -> (-115.824, -62.8583) construction
  line L15 (-115.824, -62.8583) -> (-123.444, -62.8583) construction
  line L16 (-153.924, -62.8583) -> (-153.924, -50.1583) construction
  line L17 (-153.924, -50.1583) -> (-146.304, -50.1583) construction
  line L18 (-146.304, -50.1583) -> (-146.304, -62.8583) construction
  line L19 (-146.304, -62.8583) -> (-153.924, -62.8583) construction
  line L20 (-184.404, -62.8583) -> (-184.404, -50.1583) construction
  line L21 (-184.404, -50.1583) -> (-176.784, -50.1583) construction
  line L22 (-176.784, -50.1583) -> (-176.784, -62.8583) construction
  line L23 (-176.784, -62.8583) -> (-184.404, -62.8583) construction
  line L24 (-214.884, -62.8583) -> (-214.884, -50.1583) construction
  line L25 (-214.884, -50.1583) -> (-207.264, -50.1583) construction
  line L26 (-207.264, -50.1583) -> (-207.264, -62.8583) construction
  line L27 (-207.264, -62.8583) -> (-214.884, -62.8583) construction
  line L28 (-245.364, -62.8583) -> (-245.364, -50.1583) construction
  line L29 (-245.364, -50.1583) -> (-237.744, -50.1583) construction
  line L30 (-237.744, -50.1583) -> (-237.744, -62.8583) construction
  line L31 (-237.744, -62.8583) -> (-245.364, -62.8583) construction
  point P0 (0, 0)
  point P1 (-28.194, -62.8583)
  point P2 (-58.674, -62.8583)
  point P3 (-89.154, -62.8583)
  point P4 (-119.634, -62.8583)
  point P5 (-150.114, -62.8583)
  point P6 (-180.594, -62.8583)
  point P7 (-211.074, -62.8583)
  point P8 (-241.554, -62.8583)
  point P9 (-28.194, -62.8583)
  point P10 (-58.674, -62.8583)
  point P11 (-89.154, -62.8583)
  point P12 (-119.634, -62.8583)
  point P13 (-150.114, -62.8583)
  point P14 (-180.594, -62.8583)
  point P15 (-211.074, -62.8583)
  point P16 (-241.554, -62.8583)
  dimension "d246" = 7.62
  dimension "d247" = 12.7
  constraints: 14 equal length, 8 coincident, 8 midpoint, 1 horizontal, 16 other
  measures "d246" distance of L0.start L0.end
  measures "d247" distance of L2.end L0.start
extrude "Ex: base" add sketch "Sketch:MP:base" against normal blind 4.572
extrude "Ex: fSens header pins" cut sketch "Sketch:MP:fSens header pins" against normal through all contours L34 L35 L36 L37
extrude "Ex: fSens bottom groove" cut sketch "Sketch:MP:fSens bottom groove" against normal blind 1.143 from surface at 0
extrude "Ex: for PCB headers" cut sketch "Sketch:MP:fSens header pins" along normal blind 2.54 from surface at -4.572
extrude "Ex: fSens front wall" add sketch "Sketch:MP:fSens front wall" along normal blind 7.62
hole "Hole: fSens 4-40 thread insert" at (29.2169, -18.6715, 0) at (29.2169, -32.6415, 0) direction (0, 0, -1) diameter 4.445 end through all
pattern_linear "Rectangular Pattern1" count 8 spacing 30.48 along (1, 0, 0) of "Ex: fSens header pins", "Ex: fSens bottom groove", "Hole: fSens 4-40 thread insert", "Ex: for PCB headers", "Ex: fSens front wall"
extrude "Ex: extend top to MM screws" add sketch "Sketch:MP: MM screws" against normal blind 4.572
extrude "Ex: extend top cut flush to MM" cut sketch "Sketch:MP: MM screws" against normal blind 0.7366
hole "Hole: MM screws: 4-40 through hole" at (96.52, 9.0678, 0) at (157.48, 9.0678, 0) at (218.44, 9.0678, 0) direction (0, 0, -1) diameter 3.556 end through all both
extrude "Ex: numbers: front" cut sketch "Sketch:MP:numbers_front" against normal blind 0.508
extrude "Ex: numbers: back" [suppressed]
fillet "Fillet1" radius 0.635 8 edges at (15.6279, -24.0665, 7.62) (46.1079, -24.0665, 7.62) (76.5879, -24.0665, 7.62) (107.0679, -24.0665, 7.62) (137.5479, -24.0665, 7.62) (168.0279, -24.0665, 7.62) (198.5079, -24.0665, 7.62) (228.9879, -24.0665, 7.62)
fillet "Fillet2" radius 2.54 16 edges at (47.1874, -8.8265, 0) (16.7074, -8.8265, 0) (16.7074, -39.3065, 0) (47.1874, -39.3065, 0) (77.6674, -39.3065, 0) (108.1474, -39.3065, 0) (138.6274, -39.3065, 0) (169.1074, -39.3065, 0) (199.5874, -39.3065, 0) (230.0674, -39.3065, 0) (169.1074, -8.8265, 0) (199.5874, -8.8265, 0) (230.0674, -8.8265, 0) (138.6274, -8.8265, 0) (108.1474, -8.8265, 0) (77.6674, -8.8265, 0)
fillet "Fillet3" radius 0.635 64 edges at (46.1079, -8.8265, 4.7625) (46.2939, -8.8265, 7.434) (47.5049, -8.8265, 7.62) (46.1079, -8.0826, 0.7439) (46.2939, -39.3065, 7.434) (47.5049, -39.3065, 7.62) (46.1079, -40.0504, 0.7439) (46.1079, -39.3065, 4.7625) (76.5879, -8.8265, 4.7625) (76.7739, -8.8265, 7.434) (77.9849, -8.8265, 7.62) (76.5879, -8.0826, 0.7439) (76.7739, -39.3065, 7.434) (77.9849, -39.3065, 7.62) (76.5879, -40.0504, 0.7439) (76.5879, -39.3065, 4.7625) (107.2539, -8.8265, 7.434) (108.4649, -8.8265, 7.62) (107.0679, -8.0826, 0.7439) (107.0679, -8.8265, 4.7625) (137.7339, -8.8265, 7.434) (138.9449, -8.8265, 7.62) (137.5479, -8.0826, 0.7439) (137.5479, -8.8265, 4.7625) (168.2139, -8.8265, 7.434) (169.4249, -8.8265, 7.62) (168.0279, -8.0826, 0.7439) (168.0279, -8.8265, 4.7625) (198.6939, -8.8265, 7.434) (199.9049, -8.8265, 7.62) (198.5079, -8.0826, 0.7439) (198.5079, -8.8265, 4.7625) (229.1739, -8.8265, 7.434) (230.3849, -8.8265, 7.62) (228.9879, -8.0826, 0.7439) (228.9879, -8.8265, 4.7625) (15.8139, -8.8265, 7.434) (17.0249, -8.8265, 7.62) (15.6279, -8.0826, 0.7439) (15.6279, -8.8265, 4.7625) (15.8139, -39.3065, 7.434) (17.0249, -39.3065, 7.62) (15.6279, -40.0504, 0.7439) (15.6279, -39.3065, 4.7625) (107.2539, -39.3065, 7.434) (108.4649, -39.3065, 7.62) (107.0679, -40.0504, 0.7439) (107.0679, -39.3065, 4.7625) (137.7339, -39.3065, 7.434) (138.9449, -39.3065, 7.62) (137.5479, -40.0504, 0.7439) (137.5479, -39.3065, 4.7625) (168.2139, -39.3065, 7.434) (169.4249, -39.3065, 7.62) (168.0279, -40.0504, 0.7439) (168.0279, -39.3065, 4.7625) (198.6939, -39.3065, 7.434) (199.9049, -39.3065, 7.62) (198.5079, -40.0504, 0.7439) (198.5079, -39.3065, 4.7625) (229.1739, -39.3065, 7.434) (230.3849, -39.3065, 7.62) (228.9879, -40.0504, 0.7439) (228.9879, -39.3065, 4.7625)
fillet "Fillet4" radius 0.635 24 edges at (76.5879, -24.0665, 0) (107.0679, -24.0665, 0) (137.5479, -24.0665, 0) (168.0279, -24.0665, 0) (198.5079, -24.0665, 0) (228.9879, -24.0665, 0) (15.6279, -24.0665, 0) (46.3123, -7.2264, 0) (46.3123, -40.9066, 0) (46.1079, -24.0665, 0) (76.7923, -7.2264, 0) (76.7923, -40.9066, 0) (107.2723, -7.2264, 0) (107.2723, -40.9066, 0) (137.7523, -7.2264, 0) (137.734, -40.8572, 0) (168.2323, -7.2264, 0) (168.2323, -40.9066, 0) (198.7123, -7.2264, 0) (198.7123, -40.9066, 0) (229.1923, -7.2264, 0) (229.1923, -40.9066, 0) (15.8323, -7.2264, 0) (15.814, -40.8572, 0)
hole "Hole: VH screws" at (158.115, -91.8972, 0) at (97.155, -91.8972, 0) at (36.195, -91.8972, 0) at (219.075, -91.8972, 0) direction (0, 0, -1) diameter 4.191 end through all
sketch "Sketch31" plane through (0, 0, 0) normal (0, 0, 1) x (1, 0, 0)
  line L0 (15.113, -5.0292) -> (244.113, -5.0292)
  line L1 (244.113, -5.0292) -> (244.113, -96.3422)
  line L2 (244.113, -96.3422) -> (15.113, -96.3422)
  line L3 (15.113, -96.3422) -> (15.113, -5.0292)
  line L4 (244.113, -5.0292) -> (248.539, -5.0292)
  line L5 (248.539, -5.0292) -> (248.539, -96.3422)
  line L6 (248.539, -96.3422) -> (244.113, -96.3422)
  line L7 (248.539, -5.0292) -> (15.113, -5.0292) projected
  line L8 (15.113, -96.3422) -> (248.539, -96.3422) projected
  point P0 (0, 0)
  dimension "d300" = 229
  constraints: 14 end point, 2 coincident, 2 point on line, 1 perpendicular
  measures "d300" distance between parallel lines of L3 L1
extrude "cut to fit build plate" cut sketch "Sketch31" along normal through all both and the other way through all contours L4 L5 L6 L1
sketch "Sketch:MP: PCB holes" plane through (0, 0, -4.572) normal (0, 0, -1) x (-1, 0, 0)
  circle A0 centre (-205.1731, -101.619) radius 1.6383
  circle A1 centre (-205.1731, -43.199) radius 1.6383
  circle A2 centre (-88.3331, -43.199) radius 1.6383
  circle A3 centre (-88.3331, -101.619) radius 1.6383
  point P0 (0, 0)
  constraints: 4 centre point, 8 other
hole "Hole: for mounting PCB" [suppressed]
equation "\"distance_to_clear_MM_and_MMC\" = 7.4422"
body "Solid1"
